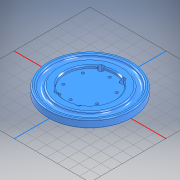
# Autodesk Inventor part: 000.005.001.002 - Поворотное основание
Saved by Autodesk Inventor 2022 (Build 260153000, 153)
## iProperties
Created: 2022-11-17
Part Number: 000.005.001.002 - Поворотное основание
Material: Пластик АБС
Document SubType Name: Modeling
Designer: Petrov Ivan
Density: 1.06 g/cm^3
Appearance: Голубой
Author: Petrov Ivan
Autodesk Inventor part; units mm, degrees
ref_plane "YZ Plane" through (0, 0, 0) normal (1, 0, 0) x (0, 1, 0)
ref_plane "XZ Plane" through (0, 0, 0) normal (0, 1, 0) x (-1, 0, 0)
ref_plane "XY Plane" through (0, 0, 0) normal (0, 0, 1) x (1, 0, 0)
sketch "Эскиз1" plane through (0, 0, 0) normal (0, 1, 0) x (-1, 0, 0)
  circle A0 centre (0, 0) radius 77.5
  dimension "d0" = 155
  constraints: 1 centre point, 1 coincident
  measures "d0" diameter of A0
extrude "Выдавливание1" add sketch "Эскиз1" along normal blind 15
sketch "Эскиз2" plane through (0, 15, 0) normal (0, 1, 0) x (1, 0, 0)
  circle A0 centre (0, 0) radius 70 construction
  circle A1 centre (0, 0) radius 60 construction
  circle A2 centre (0, 0) radius 65
  dimension "d7" = 140
  dimension "d6" = 120
  dimension "d5" = 130
  constraints: 3 centre point, 3 coincident
  measures "d7" diameter of A0
  measures "d6" diameter of A1
  measures "d5" diameter of A2
sketch "Эскиз3" plane through (0, 0, 0) normal (0, 0, 1) x (1, 0, 0)
  line L0 (65, 15) -> (-65, 15) projected
  circle A0 centre (-65, 15) radius 5.15
  point P0 (0, 0)
  dimension "d8" = 10.3
  constraints: 1 centre point, 1 coincident
  measures "d8" diameter of A0
sweep "Сдвиг1" cut profiles "Эскиз3" path "Эскиз2"
fillet "Сопряжение1" radius 3 2 edges at (-70.15, 15, 0) (-59.85, 15, 0)
fillet "Сопряжение2" radius 2 2 edges at (77.5, 15, 0) (77.5, 0, 0)
sketch "Эскиз4" plane through (0, 15, 0) normal (0, 1, 0) x (1, 0, 0)
  circle A0 centre (0, 0) radius 14 construction
  circle A1 centre (0, 0) radius 45
  dimension "d11" = 28
  dimension "d12" = 90
  constraints: 2 centre point, 2 coincident
  measures "d11" diameter of A0
  measures "d12" diameter of A1
extrude "Выдавливание2" cut sketch "Эскиз4" against normal blind 5
sketch "Эскиз5" plane through (0, 10, 0) normal (0, 1, 0) x (1, 0, 0)
  circle A0 centre (0, -36) radius 2.5
  point P0 (0, 0)
  dimension "d15" = 5
  dimension "d16" = 36
  constraints: 1 centre point
  measures "d15" diameter of A0
  measures "d16" distance of point (0, 0) A0.centre
extrude "Выдавливание3" cut sketch "Эскиз5" against normal through all
pattern_circular "Круговой массив1" count 6 over 360 about axis through (0, 15, 0) along (0, -1, 0) of "Выдавливание3"
chamfer "Фаска1" distance 2 angle 45 1 edges at (-45, 15, 0)
sketch "Эскиз6" plane through (0, 0, 0) normal (0, -1, 0) x (1, 0, 0)
  circle A0 centre (0, 36) radius 2.5 projected
  circle A1 centre (0, 36) radius 6
  point P0 (0, 0)
  dimension "d31" = 12
  constraints: 1 centre point, 1 coincident
  measures "d31" diameter of A1
extrude "Выдавливание4" cut sketch "Эскиз6" against normal blind 5
pattern_circular "Круговой массив2" count 6 over 360 about axis through (0, 0, 0) along (0, 1, 0) of "Выдавливание4"
sketch "Эскиз7" plane through (0, 0, 0) normal (0, -1, 0) x (1, 0, 0)
  circle A0 centre (20, 40) radius 2.5
  point P0 (0, 0)
  dimension "d37" = 5
  dimension "d40" = 40
  dimension "d41" = 20
  constraints: 1 centre point
  measures "d37" diameter of A0
  measures "d40" vertical distance of point (0, 0) A0.centre
  measures "d41" horizontal distance of point (0, 0) A0.centre
extrude "Выдавливание5" cut sketch "Эскиз7" against normal through all
sketch "Эскиз8" plane through (0, 10, 0) normal (0, 1, 0) x (1, 0, 0)
  arc A0 (22.3219, -39.0734) -> (17.8656, -41.3016) centre (20, -40) ccw projected
  line L0 (15.0925, -40) -> (17.5463, -35.75)
  line L1 (17.5463, -35.75) -> (22.4537, -35.75)
  line L2 (22.4537, -35.75) -> (24.9075, -40)
  line L3 (24.9075, -40) -> (22.4537, -44.25)
  line L4 (22.4537, -44.25) -> (17.5463, -44.25)
  line L5 (17.5463, -44.25) -> (15.0925, -40)
  point P0 (0, 0)
  dimension "d42" = 8.5
  constraints: 12 end point, 1 coincident, 13 other
  measures "d42" distance between parallel lines of L4 L1
extrude "Выдавливание6" cut sketch "Эскиз8" along normal mid plane 14
mirror "Зеркальное отражение1" about plane through (0, 0, 0) normal (0, 0, 1) of "Выдавливание6", "Выдавливание5"
mirror "Зеркальное отражение2" about plane through (0, 0, 0) normal (1, 0, 0) of "Выдавливание6", "Выдавливание5", "Зеркальное отражение1"
sketch "Эскиз9" plane through (0, 0, 0) normal (0, -1, 0) x (1, 0, 0)
  circle A0 centre (0, 0) radius 77.5 projected
  circle A1 centre (20, 40) radius 2.5 projected
  circle A2 centre (-20, 40) radius 2.5 projected
  circle A3 centre (-20, -40) radius 2.5 projected
  circle A4 centre (20, -40) radius 2.5 projected
equation "\"d5\" = 0.5 * d6 + 0.5 * d7"
